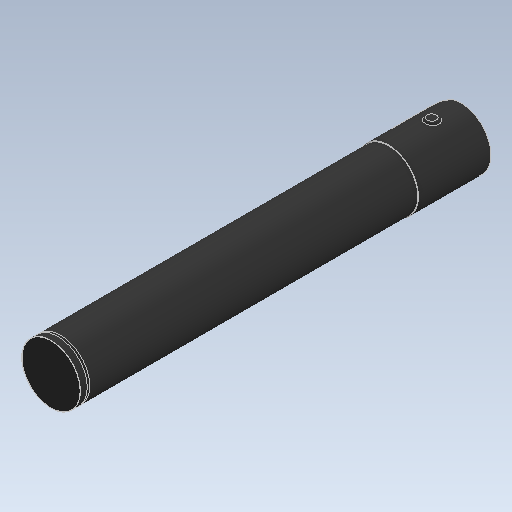
# Autodesk Inventor part: LAIRD_001-0012_Upper
Saved by Autodesk Inventor 2021 (Build 250183000, 183)
## iProperties
Created: 2020-06-10
Part Number: LAIRD_001-0012_Upper
Material: Generic
Document SubType Name: Modeling
Designer: lgnds
Density: 1 g/cm^3
Appearance: Default
Author: lgnds
Autodesk Inventor part; units mm, degrees
ref_plane "YZ Plane" through (0, 0, 0) normal (1, 0, 0) x (0, 1, 0)
ref_plane "XZ Plane" through (0, 0, 0) normal (0, 1, 0) x (-1, 0, 0)
sketch "Sketch1" plane through (0, 0, 0) normal (0, 0, 1) x (1, 0, 0)
  circle A0 centre (0, 0) radius 6.6
  dimension "d0" = 13.2
  constraints: 1 centre point, 1 coincident
  measures "d0" diameter of A0
extrude "Extrusion1" add sketch "Sketch1" along normal blind 89.9
ref_plane "Work Plane1" through (0, 0, 88.4) normal (0, 0, 1) x (1, 0, 0)
sketch "Sketch2" plane through (0, 0, 88.4) normal (0, 0, 1) x (1, 0, 0)
  circle A0 centre (0, 0) radius 6.6 projected
  circle A1 centre (0, 0) radius 6.1
  dimension "d4" = 0.5
  constraints: 1 centre point, 1 coincident
  measures "d4" radial gap between concentric circles of A0 A1
extrude "Extrusion2" cut sketch "Sketch2" against normal blind 0.2
fillet "Fillet1" radius 1 1 edges at (-6.6, 0, 88.2)
fillet "Fillet2" radius 0.2 1 edges at (-6.6, 0, 89.9)
sketch "Sketch3" plane through (0, 0, 0) normal (0, 1, 0) x (-1, 0, 0)
  line L0 (6.6, 0) -> (-6.6, 0) projected
  line L1 (6.6, 87.334) -> (-6.6, 87.334) projected
  line L2 (6.6, 0) -> (6.6, 87.334) projected
  line L3 (6.6, 12) -> (4.6, 10)
  line L4 (4.6, 10) -> (4.6, 1.0698)
  line L5 (4.6, 1.0698) -> (1.6608, 0)
  line L6 (6.6, 0) -> (-6.6, 0) projected
  line L7 (1.6608, 0) -> (6.6, 0)
  line L8 (6.6, 12) -> (6.6, 0)
  point P0 (0, 0)
  dimension "d9" = 12
  dimension "d10" = 45
  dimension "d11" = 2
  dimension "d12" = 20
  constraints: 10 end point, 2 point on line, 1 collinear, 1 vertical
  measures "d9" distance from line of L0 L3.start
  measures "d10" angle of L2 L3
  measures "d11" distance between parallel lines of L2 L4
  measures "d12" angle of L5 L0
extrude "Extrusion3" cut sketch "Sketch3" along normal through all both and the other way through all
sketch "Sketch4" plane through (0, 0, 89.9) normal (0, 0, 1) x (1, 0, 0)
  circle A0 centre (0, 0) radius 6.45
  circle A1 centre (0, 0) radius 6.6 projected
  dimension "d15" = 12.9
  constraints: 1 centre point, 1 coincident
  measures "d15" diameter of A0
extrude "Extrusion4" cut sketch "Sketch4" against normal blind 74
sketch "Sketch5" plane through (0, 0, 0) normal (0, 0, -1) x (-1, 0, 0)
  circle A0 centre (0, 0) radius 5.6
  arc A1 (1.6608, 6.3876) -> (1.6608, -6.3876) centre (0, 0) ccw projected
  dimension "d18" = 1
  constraints: 1 centre point, 1 coincident
  measures "d18" radial gap between concentric circles of A1 A0
extrude "Extrusion5" cut sketch "Sketch5" against normal up to surface (15.9 mm away)
sketch "Sketch6" plane through (0, 0, 0) normal (0, 1, 0) x (-1, 0, 0)
  line L0 (0, -17.98) -> (0, 107.88) projected
  circle A0 centre (0, 6.35) radius 1.5
  line L1 (1.6608, 0) -> (-6.6, 0) projected
  point P0 (0, 0)
  dimension "d21" = 6.35
  dimension "d22" = 3
  constraints: 1 centre point, 1 point on line
  measures "d21" distance from line of L1 A0.centre
  measures "d22" diameter of A0
extrude "Extrusion6" add sketch "Sketch6" along normal mid plane 14
fillet "Fillet3" radius 0.5 2 edges at (1.5, 7, 6.35) (1.5, -7, 6.35)
fillet "Fillet4" radius 3 4 edges at (-4.6, 3.9633, 1.0698) (-4.6, -3.9633, 1.0698) (-1.6608, -5.8679, 0) (-1.6608, 5.8679, 0)
body "Solid1"
